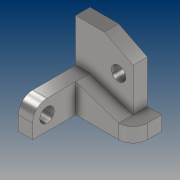
# Autodesk Inventor part: 30
Saved by Autodesk Inventor 2020.2 (Build 242310000, 310)
## iProperties
Created: 2020-09-17
Part Number: 30
Material: 鋼、碳鋼
Document SubType Name: Modeling
Designer: user
Density: 7.85 g/cm^3
Appearance: 半拋光
Mass: 247.275 g
Surface Area: 91.8231 cm^2
Volume: 31.5 cm^3
Author: user
Autodesk Inventor part; units mm, degrees
ref_plane "YZ Plane" through (0, 0, 0) normal (1, 0, 0) x (0, 1, 0)
ref_plane "XZ Plane" through (0, 0, 0) normal (0, 1, 0) x (-1, 0, 0)
ref_plane "XY Plane" through (0, 0, 0) normal (0, 0, 1) x (1, 0, 0)
sketch "草圖1" plane through (0, 0, 0) normal (0, 1, 0) x (-1, 0, 0)
  line L0 (0, 0) -> (-50, 0)
  line L1 (-50, 0) -> (-50, 20)
  line L2 (-50, 20) -> (0, 20)
  line L3 (0, 20) -> (0, 0)
  line L4 (0, 0) -> (-10, 0)
  line L5 (-10, 0) -> (-10, 50)
  line L6 (-10, 50) -> (0, 50)
  line L7 (0, 50) -> (0, 0)
  dimension "d0" = 50
  dimension "d1" = 20
  dimension "d2" = 50
  dimension "d3" = 10
  constraints: 16 end point, 4 parallel, 2 horizontal, 2 perpendicular
  measures "d0" distance of L0.start L0.end
  measures "d1" distance of L0.end L1.end
  measures "d2" distance of L6.end L0.start
  measures "d3" distance of L5.end L6.end
extrude "擠出1" add sketch "草圖1" along normal blind 20 contours L0 L5 L2 L3 | L2 L5 L6 L7
extrude "擠出2" add sketch "草圖1" along normal blind 50 contours L0 L5 L2 L3 | L0 L1 L2 L5
sketch "草圖3" plane through (0, 50, 0) normal (0, 1, 0) x (1, 0, 0)
  line L0 (50, -20) -> (0, -20) projected
  line L1 (0, -20) -> (0, 0) projected
  line L2 (0, 0) -> (50, 0) projected
  line L3 (0, -20) -> (10, -20)
  line L4 (10, -20) -> (10, -10)
  line L5 (10, -10) -> (0, -10)
  line L6 (0, -10) -> (0, -20)
  line L7 (10, -50) -> (10, -20) projected
  line L8 (50, 0) -> (50, -20) projected
  point P0 (0, -10)
  dimension "d12" = 10
  constraints: 8 end point, 2 parallel, 1 collinear, 1 horizontal, 1 perpendicular
  measures "d12" distance of L3.end L4.end
extrude "擠出4" cut sketch "草圖3" against normal up to surface (30 mm away) contours L0 L1 L5 L4
sketch "草圖4" plane through (0, 50, 0) normal (0, 1, 0) x (1, 0, 0)
  line L0 (50, -20) -> (10, -20) projected
  line L1 (10, -20) -> (10, -10) projected
  line L2 (10, -10) -> (0, -10) projected
  line L3 (0, -10) -> (0, 0) projected
  line L4 (0, 0) -> (50, 0) projected
  line L5 (10, -10) -> (10, -20) projected
  line L6 (10, -10) -> (63.9282, -10)
  line L7 (63.9282, -10) -> (63.9282, -20)
  line L8 (63.9282, -20) -> (10, -20)
  line L9 (10, -20) -> (10, -10)
  line L10 (10, -20) -> (50, -20) projected
  line L11 (50, 0) -> (50, -20) projected
  point P0 (30, -20)
  constraints: 8 end point, 2 parallel, 1 collinear, 1 horizontal, 1 perpendicular
extrude "擠出5" cut sketch "草圖4" against normal blind 30 contours L11 L6 L7 L8 | L0 L1 L6 L11
sketch "草圖5" plane through (10, 0, 20) normal (0, 0, 1) x (1, 0, 0)
  line L0 (40, 20) -> (40, 0) projected
  line L1 (40, 0) -> (0, 0) projected
  line L2 (0, 0) -> (-10, 0) projected
  line L3 (-10, 0) -> (-10, 20) projected
  line L4 (-10, 20) -> (0, 20) projected
  line L5 (0, 20) -> (40, 20) projected
  line L6 (0, 20) -> (0, 0) projected
  line L7 (0, 20) -> (30, 10)
  line L8 (30, 10) -> (40, 10)
  line L9 (40, 0) -> (40, 50) projected
  dimension "d17" = 10
  dimension "d18" = 10
  constraints: 4 end point, 1 horizontal, 1 point on line
  measures "d17" distance between parallel lines of L8 L1
  measures "d18" distance of L7.end L8.end
extrude "擠出6" cut sketch "草圖5" against normal blind 10 contours L0 L8 L7 L5
sketch "草圖6" plane through (0, 50, 10) normal (0, 0, 1) x (1, 0, 0)
  line L0 (0, -50) -> (0, -30) projected
  line L1 (0, -30) -> (0, 0) projected
  line L2 (0, 0) -> (50, 0) projected
  line L3 (50, 0) -> (50, -40) projected
  line L4 (50, -40) -> (50, -50) projected
  line L5 (50, -50) -> (0, -50) projected
  line L6 (0, -30) -> (10, -30) projected
  line L7 (10, -30) -> (40, -40) projected
  line L8 (40, -40) -> (50, -40) projected
  line L9 (0, 0) -> (50, 0) projected
  line L10 (40, -40) -> (50, -40)
  line L11 (50, -40) -> (50, 0)
  line L12 (50, 0) -> (40, 0)
  line L13 (40, 0) -> (40, -40)
  line L14 (40, -10) -> (20, 0)
  point P0 (20, 0)
  dimension "d21" = 20
  dimension "d22" = 10
  constraints: 10 end point, 2 parallel, 2 point on line, 1 horizontal, 1 perpendicular
  measures "d21" distance from line of L14.end L13
  measures "d22" distance from line of L14.start L2
extrude "擠出7" cut sketch "草圖6" against normal blind 10 contours L8 L13 L2 L3 | L2 L13 L14
fillet "圓角1" radius 10 1 edges at (50, 5, 20)
fillet "圓角2" radius 10 1 edges at (5, 20, 50)
sketch "草圖7" plane through (0, 20, 10) normal (0, 0, 1) x (1, 0, 0)
  line L0 (20, 30) -> (40, 20) projected
  line L1 (40, 20) -> (40, -10) projected
  line L2 (40, -10) -> (50, -10) projected
  line L3 (50, -10) -> (50, -20) projected
  line L4 (50, -20) -> (0, -20) projected
  line L5 (0, -20) -> (0, 0) projected
  line L6 (0, 0) -> (0, 30) projected
  line L7 (0, 30) -> (20, 30) projected
  line L8 (10, 0) -> (40, -10) projected
  line L9 (0, 0) -> (10, 0) projected
  point P0 (30, 10)
  dimension "d27" = 10
  dimension "d28" = 20
  measures "d27" distance from line of L1 point (30, 10)
  measures "d28" distance from line of L7 point (30, 10)
hole "孔1" at (30, 30, 10) direction (0, 0, -1) diameter 10 end through all
sketch "草圖8" plane through (10, 0, 50) normal (1, 0, 0) x (0, 0, -1)
  arc A0 (10, 20) -> (0, 10) centre (10, 10) ccw projected
  point P0 (50, 0)
  constraints: 1 coincident
hole "孔2" at (10, 10, 40) direction (-1, 0, 0) diameter 10 end through all
